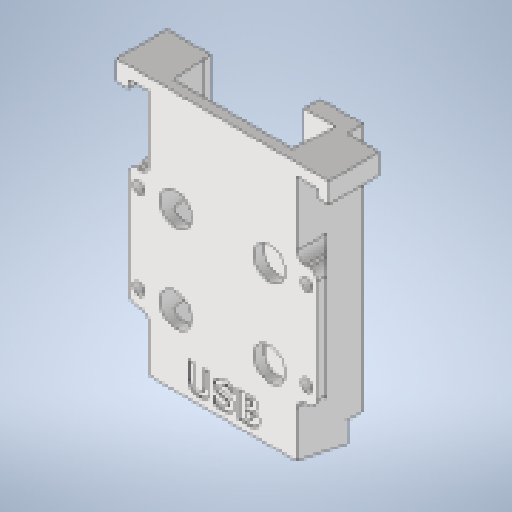
# Autodesk Inventor part: TPLink_holder
Saved by Autodesk Inventor 2025.1 (Build 291241000, 241)
## iProperties
Created: 2026-04-16
Part Number: TPLink_holder
Material: Generic
Document SubType Name: Modeling
Designer: User
Density: 1 g/cm^3
Appearance: Default
Author: User
## iProperties of the stored document TPLink_holder_3DPrint.ipt
Created: 2026-04-16
Part Number: TPLink_holder_3DPrint
Material: Generic
Document SubType Name: Modeling
Designer: User
Density: 1 g/cm^3
Appearance: Default
Author: User
Autodesk Inventor part; units mm, degrees
ref_plane "YZ Plane" through (0, 0, 0) normal (1, 0, 0) x (0, 1, 0)
ref_plane "XZ Plane" through (0, 0, 0) normal (0, 1, 0) x (-1, 0, 0)
ref_plane "XY Plane" through (0, 0, 0) normal (0, 0, 1) x (1, 0, 0)
sketch "Sketch1" plane through (0, 0, 0) normal (0, 0, 1) x (1, 0, 0)
  circle A0 centre (-2.95, 14.395506) radius 1.5
  circle A1 centre (-2.95, -16.594833) radius 1.5
  circle A2 centre (-31.617451, -2.998229) radius 1.5
  arc A3 (-69.05, 18.492691) -> (-67.05, 16.492691) centre (-67.05, 18.492691) ccw
  line L0 (-69.05, 18.492691) -> (-69.05, 32.5)
  line L1 (-69.05, 32.5) -> (-72.05, 32.5)
  line L2 (-72.05, -34) -> (-72.05, 32.5)
  line L3 (-72.05, -34) -> (-69.05, -34)
  line L4 (-69.05, -34) -> (-69.05, -28.3)
  arc A4 (-67.05, -26.3) -> (-69.05, -28.3) centre (-67.05, -28.3) ccw
  line L5 (-67.05, -26.3) -> (-43.236448, -26.3)
  arc A5 (-43.236448, -26.3) -> (-41.236448, -24.3) centre (-43.236448, -24.3) ccw
  line L6 (-41.236448, -24.3) -> (-41.236448, -18.699925)
  arc A6 (-39.236448, -16.699925) -> (-41.236448, -18.699925) centre (-39.236448, -18.699925) ccw
  line L7 (-39.236448, -16.699925) -> (-25.536448, -16.699925)
  arc A7 (-23.536448, -18.699925) -> (-25.536448, -16.699925) centre (-25.536448, -18.699925) ccw
  line L8 (-23.536448, -18.699925) -> (-23.536448, -24.3)
  arc A8 (-23.536448, -24.3) -> (-21.536448, -26.3) centre (-21.536448, -24.3) ccw
  line L9 (-21.536448, -26.3) -> (16.15, -26.3)
  line L10 (16.15, -26.3) -> (16.15, -32)
  line L11 (16.15, -32) -> (19.15, -32)
  line L12 (19.15, -32) -> (19.15, -23)
  line L13 (19.15, -23) -> (11.85, -23)
  line L14 (5.85, -17) -> (11.85, -23)
  line L15 (5.85, -17) -> (5.85, -14.65)
  arc A9 (5.85, -14.65) -> (3.85, -12.65) centre (3.85, -14.65) ccw
  line L16 (3.85, -12.65) -> (-0.35, -12.65)
  arc A10 (-2.35, -10.65) -> (-0.35, -12.65) centre (-0.35, -10.65) ccw
  line L17 (-2.35, -10.65) -> (-2.35, 10.65)
  arc A11 (-0.35, 12.65) -> (-2.35, 10.65) centre (-0.35, 10.65) ccw
  line L18 (-0.35, 12.65) -> (3.85, 12.65)
  arc A12 (3.85, 12.65) -> (5.85, 14.65) centre (3.85, 14.65) ccw
  line L19 (5.85, 14.65) -> (5.85, 17)
  line L20 (11.85, 23) -> (5.85, 17)
  line L21 (11.85, 23) -> (19.15, 23)
  line L22 (19.15, 23) -> (19.15, 32)
  line L23 (19.15, 32) -> (16.15, 32)
  line L24 (16.15, 32) -> (16.15, 24.50333)
  line L25 (16.15, 24.50333) -> (11.05, 24.50333)
  line L26 (11.05, 24.50333) -> (11.05, 25.3)
  line L27 (11.05, 25.3) -> (-13.742981, 25.3)
  arc A13 (-13.742981, 25.3) -> (-15.742981, 23.3) centre (-13.742981, 23.3) ccw
  line L28 (-15.742981, 23.3) -> (-15.742981, 17.729975)
  arc A14 (-17.742981, 15.729975) -> (-15.742981, 17.729975) centre (-17.742981, 17.729975) ccw
  line L29 (-17.742981, 15.729975) -> (-38.743552, 15.729975)
  arc A15 (-40.743552, 17.729975) -> (-38.743552, 15.729975) centre (-38.743552, 17.729975) ccw
  line L30 (-40.743552, 17.729975) -> (-40.743552, 23.3)
  arc A16 (-40.743552, 23.3) -> (-42.743552, 25.3) centre (-42.743552, 23.3) ccw
  line L31 (-42.743552, 25.3) -> (-50.436553, 25.3)
  arc A17 (-50.436553, 25.3) -> (-52.436553, 23.3) centre (-50.436553, 23.3) ccw
  line L32 (-52.436553, 23.3) -> (-52.436553, 18.492691)
  arc A18 (-54.436553, 16.492691) -> (-52.436553, 18.492691) centre (-54.436553, 18.492691) ccw
  line L33 (-54.436553, 16.492691) -> (-67.05, 16.492691)
  line L34 (-6.107274, -23.520089) -> (-6.107274, 44.519148)
  ellipse E0 centre (-12.125904, -23.420884) end of major axis (-9.966677, -29.178822) minor radius 6 (-12.028521, -29.552133) -> (-6.107274, -23.520089) ccw
  line L35 (-30.786028, -29.552133) -> (-12.028521, -29.552133)
  ellipse E1 centre (-30.688645, -23.420884) end of major axis (-32.847872, -29.178822) minor radius 6 (-36.707274, -23.520089) -> (-30.786028, -29.552133) ccw
  line L36 (-36.707274, 44.519148) -> (-36.707274, -23.520089)
  line L37 (-36.707274, -16.699925) -> (-36.707274, -14.699925)
  line L38 (-36.707274, -14.699925) -> (-6.107274, -14.699925)
  line L39 (-36.707274, 15.729975) -> (-36.707274, 13.729975)
  line L40 (-36.707274, 13.729975) -> (-6.107274, 13.729975)
  line L41 (-36.707274, -14.699925) -> (-6.107274, 13.729975)
  line L42 (-36.707274, 13.729975) -> (-6.107274, -14.699925)
  line L43 (-36.707274, -14.699925) -> (-33.044239, -11.296666)
  line L44 (-36.707274, 13.729975) -> (-33.044239, 10.326716)
  line L45 (-6.107274, -14.699925) -> (-9.77031, -11.296666)
  line L46 (-6.107274, 13.729975) -> (-9.77031, 10.326716)
  circle A19 centre (-9.77031, -11.296666) radius 1.5
  circle A20 centre (-9.77031, 10.326716) radius 1.5
  circle A21 centre (-33.044239, 10.326716) radius 1.5
  circle A22 centre (-33.044239, -11.296666) radius 1.5
  point P0 (0, 0)
  dimension "d0" = 2
  dimension "d1" = 90
  dimension "d2" = 2
  dimension "d3" = 5
  dimension "d4" = 5
  dimension "d5" = 5
  dimension "d6" = 5
  dimension "d7" = 3
  dimension "d8" = 3
  dimension "d9" = 3
  dimension "d10" = 3
  constraints: 20 end point, 13 point on line, 4 centre point, 3 coincident, 2 perpendicular, 2 other
  measures "d0" distance of L37.start L37.end
  measures "d1" angle of L37 L38
  measures "d2" distance of L39.start L39.end
  measures "d3" distance of L37.end L43.end
  measures "d4" distance of L39.end L44.end
  measures "d5" distance of L38.end L45.end
  measures "d6" distance of L40.end L46.end
  measures "d7" diameter of A19
  measures "d8" diameter of A20
  measures "d9" diameter of A21
  measures "d10" diameter of A22
extrude "Extrusion1" add sketch "Sketch1" along normal blind 4 contours A2 | L42 A21 L41 A22 L36 | L40 L41 A20 L42 A21 | L41 A22 L42 A19 L38 | L34 L42 A19 L41 A20
sketch "Sketch2" plane through (0, 0, 4) normal (0, 0, 1) x (1, 0, 0)
  circle A0 centre (-9.77031, -11.296666) radius 1.5
  circle A1 centre (-9.77031, 10.326716) radius 1.5
  circle A2 centre (-33.044239, -11.296666) radius 1.5
  circle A3 centre (-33.044239, 10.326716) radius 1.5
  circle A4 centre (-9.77031, -11.296666) radius 3.663035
  line L0 (-6.107274, -14.699925) -> (-6.107274, 13.729975)
  circle A5 centre (-9.77031, 10.326716) radius 3.677483
  circle A6 centre (-33.044239, 10.326716) radius 3.663035
  line L1 (-36.707274, 13.729975) -> (-36.707274, -14.699925)
  circle A7 centre (-33.044239, -11.296666) radius 3.663035
  line L2 (-36.707274, -14.699925) -> (-6.107274, -14.699925)
  line L3 (-6.107274, 13.729975) -> (-36.707274, 13.729975)
  point P0 (0, 0)
  point P1 (-34.399103, -14.699925)
  point P2 (-36.707274, -11.296666)
  point P3 (-34.399103, 13.729975)
  point P4 (-36.707274, 10.326716)
  point P5 (-6.107274, 10.001058)
  point P6 (-8.376858, 13.729975)
  point P7 (-6.107274, -11.296666)
  point P8 (-8.415446, -14.699925)
  constraints: 4 centre point, 4 coincident, 3 tangent
extrude "Extrusion2" cut sketch "Sketch2" against normal blind 2 contours A0 | A1 | A2 | A3 | A4 L2 | L0 L2 A4 | L2 A4 | A5 L3 L0 | L2 A7 | A7 L2 | A5 L3 L0 | A5 L3 | L2 L1 A7 | L3 A6 | A6 L3 | A6 L1 L3
sketch "Sketch3" plane through (-36.707274, -14.699925, 0) normal (-1, 0, 0) x (0, 0, 1)
  line L0 (4, 25.026641) -> (2, 25.026641)
  line L1 (2, 25.026641) -> (2, 28.4299)
  line L2 (0, 28.4299) -> (2, 28.4299)
  line L3 (0, 28.4299) -> (0, 0)
  line L4 (0, 0) -> (2, 0)
  line L5 (2, 0) -> (2, 3.403259)
  line L6 (4, 3.403259) -> (2, 3.403259)
  line L7 (4, 25.026641) -> (4, 3.403259)
  line L8 (0, 4.903259) -> (0, 1.903259)
  line L9 (4, 25.026641) -> (0, 25.026641)
  line L10 (0, 25.026641) -> (0, 3.403259)
  line L11 (0, 3.403259) -> (4, 3.403259)
  line L12 (4, 3.403259) -> (4, 25.026641)
  point P0 (0, 14.699925)
  point P1 (0, 3.403259)
  constraints: 8 end point, 2 parallel, 1 horizontal, 1 midpoint, 1 perpendicular
extrude "Extrusion3" add sketch "Sketch3" along normal blind 3
sketch "Sketch4" plane through (-6.107274, -14.699925, 0) normal (1, 0, 0) x (0, 0, -1)
  line L0 (-2, 28.4299) -> (-2, 24.700983)
  line L1 (-2, 24.700983) -> (-4, 24.700983)
  line L2 (-4, 3.403259) -> (-4, 24.700983)
  line L3 (-4, 3.403259) -> (-2, 3.403259)
  line L4 (-2, 3.403259) -> (-2, 0)
  line L5 (0, 0) -> (-2, 0)
  line L6 (0, 0) -> (0, 28.4299)
  line L7 (0, 28.4299) -> (-2, 28.4299)
  line L8 (-4, 3.403259) -> (0, 3.403259)
  line L9 (0, 3.403259) -> (0, 24.700983)
  line L10 (0, 24.700983) -> (-4, 24.700983)
  line L11 (-4, 24.700983) -> (-4, 3.403259)
  point P0 (0, 14.699925)
  constraints: 8 end point, 2 parallel, 1 horizontal, 1 perpendicular, 1 point on line
extrude "Extrusion4" add sketch "Sketch4" along normal blind 3
sketch "Sketch5" plane through (-39.707274, -11.296666, 4) normal (0, -1, 0) x (1, 0, 0)
  line L0 (3, 0) -> (3, -2) projected
  line L1 (3, 0) -> (0, 0) projected
  line L2 (0, -2) -> (0, 0) projected
  line L3 (3, -2) -> (0, -2) projected
  line L4 (33.6, 0) -> (33.6, -2) projected
  line L5 (33.6, -2) -> (36.6, -2) projected
  line L6 (36.6, 0) -> (36.6, -2) projected
  line L7 (33.6, 0) -> (36.6, 0) projected
  point P0 (39.707274, -4)
extrude "Extrusion5" add sketch "Sketch5" along normal up to surface (3.403259 mm away)
sketch "Sketch6" plane through (-6.107274, 10.001058, 4) normal (0, 1, 0) x (1, 0, 0)
  line L0 (0, 2) -> (0, 0) projected
  line L1 (0, 0) -> (3, 0) projected
  line L2 (3, 2) -> (3, 0) projected
  line L3 (0, 2) -> (3, 2) projected
  line L4 (-30.6, 0) -> (-30.6, 2) projected
  line L5 (-30.6, 2) -> (-33.6, 2) projected
  line L6 (-33.6, 0) -> (-33.6, 2) projected
  line L7 (-30.6, 0) -> (-33.6, 0) projected
  point P0 (6.107274, 4)
extrude "Extrusion6" add sketch "Sketch6" along normal up to surface (3.728917 mm away)
sketch "Sketch7" plane through (0, 0, 4) normal (0, 0, 1) x (1, 0, 0)
  line L0 (-39.707274, 13.729975) -> (-39.707274, -14.699925)
  line L1 (-3.107274, -14.699925) -> (-3.107274, 13.729975)
  line L2 (-3.107274, 13.729975) -> (-6.107274, 13.729975)
  line L3 (-3.107274, -14.699925) -> (-6.007274, -14.699925)
  line L4 (-6.007274, -14.699925) -> (-6.007274, 13.729975)
  line L5 (-6.007274, 13.729975) -> (-3.107274, 13.729975)
  line L6 (-3.107274, 13.729975) -> (-3.107274, -14.699925)
  line L7 (-39.707274, -14.699925) -> (-36.807274, -14.699925)
  line L8 (-36.807274, -14.699925) -> (-36.807274, 13.729975)
  line L9 (-36.807274, 13.729975) -> (-39.707274, 13.729975)
  line L10 (-39.707274, 13.729975) -> (-39.707274, -14.699925)
  point P0 (0, 0)
  dimension "d23" = 2.9
  dimension "d24" = 2.9
  constraints: 16 end point, 4 parallel, 2 horizontal, 2 perpendicular, 2 point on line
  measures "d23" distance of L4.end L5.end
  measures "d24" distance of L9.end L8.end
ref_plane "Work Plane1" through (-73.457274, -42.102133, 13.808489) normal (0, 0, 1) x (1, 0, 0)
extrude "Extrusion7" add sketch "Sketch7" along normal up to surface (9.808489 mm away)
sketch "Sketch8" plane through (-31.689375, -14.699925, 4) normal (0, -1, 0) x (1, 0, 0)
  line L0 (-4.267899, 9.808489) -> (-5.017899, 0.298489)
  line L1 (25.582101, 0.298489) -> (24.832101, 9.808489)
  line L2 (25.682101, 0) -> (25.682101, 9.808489)
  line L3 (-5.117899, 0) -> (-5.117899, 9.808489)
  line L4 (-4.46852, 9.808489) -> (-5.21728, 0.314213)
  line L5 (25.781482, 0.314213) -> (25.032722, 9.808489)
  line L6 (-8.017899, 9.808489) -> (-5.117899, 9.808489)
  line L7 (-5.117899, 9.808489) -> (-4.46852, 9.808489)
  line L8 (25.032722, 9.808489) -> (25.682101, 9.808489)
  point P0 (31.689375, -4)
  point P1 (25.682101, 1.574363)
  point P2 (-5.117899, 1.574363)
  dimension "d27" = 0.2
  dimension "d28" = 0.2
  constraints: 8 end point, 2 parallel, 1 collinear, 1 perpendicular
  measures "d27" distance between parallel lines of L0 L4
  measures "d28" distance between parallel lines of L1 L5
extrude "Extrusion8" add sketch "Sketch8" against normal up to surface (28.4299 mm away)
sketch "Sketch9" plane through (-3.107274, -14.699925, 13.808489) normal (0, 0, 1) x (1, 0, 0)
  line L0 (0, 0) -> (-3.549379, 0)
  line L1 (0, 28.4299) -> (0, 0)
  line L2 (0, 28.4299) -> (-3.549379, 28.4299)
  line L3 (-3.549379, 0) -> (-3.549379, 28.4299)
  line L4 (-36.6, 28.4299) -> (-33.050621, 28.4299)
  line L5 (-36.6, 0) -> (-36.6, 28.4299)
  line L6 (-33.050621, 0) -> (-36.6, 0)
  line L7 (-33.050621, 0) -> (-33.050621, 28.4299)
  point P0 (3.107274, 14.699925)
extrude "Extrusion9" add sketch "Sketch9" along normal blind 0.2
sketch "Sketch10" plane through (-3.107274, -14.699925, 14.008489) normal (0, 0, 1) x (1, 0, 0)
  line L0 (0, 0) -> (0, 28.4299) projected
  line L1 (-36.6, 28.4299) -> (-36.6, 0) projected
  line L2 (0, 0) -> (0, 28.4299) projected
  line L3 (0, 0) -> (-36.6, 0)
  line L4 (-36.6, 0) -> (-36.6, 28.4299)
  line L5 (-36.6, 28.4299) -> (0, 28.4299)
  line L6 (0, 28.4299) -> (0, 0)
  point P0 (3.107274, 14.699925)
  point P1 (-36.6, 0)
  constraints: 8 end point, 2 parallel, 1 horizontal, 1 perpendicular
extrude "Extrusion10" add sketch "Sketch10" along normal blind 2.5
sketch "Sketch11" plane through (-39.707274, -14.699925, 0) normal (-1, 0, 0) x (0, 0, 1)
  line L0 (4.298489, -14.852208) -> (13.808489, -12.852208)
  line L1 (4.339649, -15.047926) -> (13.849649, -13.047926)
  line L2 (16.508489, 28.4299) -> (16.508489, 0)
  line L3 (0, 0) -> (16.508489, 0)
  line L4 (0, -15.960576) -> (0, 0)
  line L5 (16.508489, 0) -> (16.508489, 28.4299)
  line L6 (16.508489, 11.085503) -> (16.508489, -12.488759)
  line L7 (16.508489, -12.488759) -> (0, -15.960576)
  point P0 (0, 14.699925)
  point P1 (4.339649, -15.047926)
  point P2 (13.849649, -13.047926)
  dimension "d35" = 0.2
  constraints: 8 end point, 1 collinear, 1 parallel, 1 point on line, 1 vertical
  measures "d35" distance between parallel lines of L0 L1
extrude "Extrusion11" add sketch "Sketch11" against normal up to surface surface through (-36.157895, -14.699925, 13.808489) normal (0.9969046, 0, -0.0786202)
sketch "Sketch12" plane through (-3.107274, -14.699925, 0) normal (1, 0, 0) x (0, 0, -1)
  line L0 (-16.508489, -12.488759) -> (-16.508489, 0)
  line L1 (0, -15.960576) -> (-16.508489, -12.488759)
  line L2 (0, 0) -> (0, -15.960576)
  line L3 (0, 0) -> (-16.508489, 0)
  point P0 (0, 14.699925)
extrude "Extrusion12" add sketch "Sketch12" against normal up to surface surface through (-6.007274, -14.699925, 5.574363) normal (-0.9969046, 0, -0.0786202)
sketch "Sketch13" plane through (-3.107274, -14.699925, 0) normal (1, 0, 0) x (0, 0, -1)
  line L0 (-16.508489, 28.4299) -> (-16.508489, -12.488759)
  line L1 (-14.008489, 0) -> (-14.008489, 28.4299)
  line L2 (-16.508489, -12.488759) -> (0, -15.960576)
  line L3 (-14.008489, 6.427758) -> (-14.008489, -13.014522)
  line L4 (-5.574363, 28.4299) -> (-13.808489, 28.4299)
  line L5 (-13.808489, 0) -> (-13.808489, 28.4299)
  line L6 (-14.008489, 0) -> (-13.808489, 0)
  line L7 (-16.508489, 0) -> (-14.008489, 0)
  line L8 (-16.508489, -12.488759) -> (-16.508489, 0)
  line L9 (0, -15.960576) -> (-16.508489, -12.488759)
  line L10 (0, 0) -> (0, -15.960576)
  line L11 (-5.574363, 0) -> (0, 0)
  line L12 (-5.574363, 28.4299) -> (-5.574363, 0)
  point P0 (0, 14.699925)
  constraints: 2 end point, 1 point on line, 1 vertical
extrude "Extrusion13" add sketch "Sketch13" against normal up to surface contours L7 L3 L2 L0 surface through (-36.157895, -14.699925, 13.808489) normal (0.9969046, 0, -0.0786202)
sketch "Sketch14" plane through (-31.689375, -14.699925, 4) normal (0, -1, 0) x (1, 0, 0)
  line L0 (26.12172, -4) -> (25.682101, 1.574363)
  line L1 (25.682101, 0) -> (25.682101, 1.574363)
  line L2 (25.582101, 0) -> (25.682101, 0)
  line L3 (25.582101, -2) -> (25.582101, 0)
  line L4 (25.582101, -2) -> (20.564202, -2)
  line L5 (20.564202, -2) -> (20.564202, 0)
  line L6 (0, 0) -> (20.564202, 0)
  line L7 (0, 0) -> (0, -2)
  line L8 (0, -2) -> (-5.017899, -2)
  line L9 (-5.017899, 0) -> (-5.017899, -2)
  line L10 (-5.117899, 0) -> (-5.017899, 0)
  line L11 (-5.117899, 0) -> (-5.117899, 1.574363)
  line L12 (-5.117899, 1.574363) -> (-5.557517, -4)
  line L13 (-5.557517, -4) -> (26.12172, -4)
  line L14 (-5.017899, 0) -> (-5.24206, 0)
  line L15 (25.582101, 0) -> (25.806262, 0)
  line L16 (20.564202, 0) -> (25.682101, 0)
  line L17 (-5.017899, 0) -> (2.308172, 0)
  line L18 (0, 0) -> (-5.017899, 0)
  point P0 (31.689375, -4)
  constraints: 8 end point, 3 point on line, 2 perpendicular, 1 horizontal
extrude "Extrusion14" add sketch "Sketch14" along normal up to surface contours L13 L12 L14 L10 L9 L8 L7 L6 L5 L4 L3 L2 L15 L0 | L3 L4 L5 L16 | L17 L7 L8 L9 surface through (-39.707274, -27.188684, 16.508489) normal (0, -0.9785934, 0.205803)
sketch "Sketch15" plane through (-3.107274, -14.699925, 0) normal (1, 0, 0) x (0, 0, -1)
  line L0 (-16.508489, -12.488759) -> (0, -15.960576)
  line L1 (-16.508489, -14.021572) -> (-0.308705, -17.428466)
  line L2 (-16.508489, 28.4299) -> (-16.508489, -12.488759)
  line L3 (0, -17.300075) -> (0, -8.300075)
  line L4 (0, -8.300075) -> (0, -17.493388)
  line L5 (0, -17.493388) -> (-16.508489, -14.021572)
  line L6 (-16.508489, -14.021572) -> (-16.508489, -12.488759)
  point P0 (0, 14.699925)
  point P1 (-0.308705, -17.428466)
  dimension "d44" = 1.5
  constraints: 8 end point, 2 parallel, 1 vertical
  measures "d44" distance between parallel lines of L0 L1
extrude "Extrusion15" add sketch "Sketch15" against normal blind 10
sketch "Sketch16" plane through (-39.707274, -14.699925, 0) normal (-1, 0, 0) x (0, 0, 1)
  line L0 (0, -17.493388) -> (16.508489, -14.021572)
  line L1 (16.508489, -14.021572) -> (16.508489, -12.488759)
  line L2 (14.008489, -13.014522) -> (16.508489, -12.488759)
  line L3 (14.008489, -13.014522) -> (4, -15.119356)
  line L4 (0, -15.960576) -> (4, -15.119356)
  line L5 (0, -15.960576) -> (0, -17.493388)
  point P0 (0, 14.699925)
extrude "Extrusion16" add sketch "Sketch16" against normal blind 10
sketch "Sketch17" plane through (-3.107274, -14.699925, 16.508489) normal (0, 0, 1) x (1, 0, 0)
  circle A0 centre (-6.663035, 3.403259) radius 1.5
  circle A1 centre (-29.936965, 3.403259) radius 1.5
  circle A2 centre (-29.936965, 3.403259) radius 4
  circle A3 centre (-6.663035, 3.403259) radius 4
  point P0 (3.107274, 14.699925)
  dimension "d49" = 8
  dimension "d50" = 8
  constraints: 2 centre point, 2 coincident
  measures "d49" diameter of A2
  measures "d50" diameter of A3
extrude "Extrusion17" cut sketch "Sketch17" against normal up to surface (2.5 mm away) contours A0 | A1 | A2 | A3
sketch "Sketch18" plane through (0, 0, 0) normal (0, 0, -1) x (-1, 0, 0)
  line L0 (23.536448, -18.699925) -> (23.536448, -24.3)
  arc A0 (21.536448, -26.3) -> (23.536448, -24.3) centre (21.536448, -24.3) ccw
  arc A1 (25.536448, -16.699925) -> (23.536448, -18.699925) centre (25.536448, -18.699925) ccw
  line L1 (39.236448, -16.699925) -> (25.536448, -16.699925)
  arc A2 (41.236448, -18.699925) -> (39.236448, -16.699925) centre (39.236448, -18.699925) ccw
  line L2 (21.536448, -26.3) -> (-16.15, -26.3)
  line L3 (39.707274, -32.193313) -> (29.707274, -32.193313)
  line L4 (39.707274, 13.729975) -> (39.707274, -32.193313)
  line L5 (29.707274, -30.660501) -> (13.107274, -30.660501)
  line L6 (29.707274, -32.193313) -> (29.707274, -30.660501)
  line L7 (13.107274, -30.660501) -> (13.107274, -32.193313)
  line L8 (3.107274, -32.193313) -> (13.107274, -32.193313)
  line L9 (3.107274, -32.193313) -> (3.107274, 13.729975)
  point P0 (0, 0)
  point P1 (3.107274, -26.3)
  point P2 (39.707274, -16.756134)
extrude "Extrusion18" cut sketch "Sketch18" against normal up to surface (4 mm away)
sketch "Sketch19" plane through (-39.707274, 13.729975, 0) normal (0, 1, 0) x (1, 0, 0)
  line L0 (3.549379, -13.808489) -> (3.549379, -14.008489)
  line L1 (2.9, -5.574363) -> (3.549379, -13.808489)
  line L2 (2.9, -4) -> (2.9, -5.574363)
  line L3 (3, -4) -> (2.9, -4)
  line L4 (3, -2) -> (3, -4)
  line L5 (8.017899, -2) -> (3, -2)
  line L6 (8.017899, -2) -> (8.017899, -4)
  line L7 (28.543513, -4) -> (8.017899, -4)
  line L8 (28.543513, -4) -> (28.543513, -2)
  line L9 (28.543513, -2) -> (33.6, -2)
  line L10 (33.6, -4) -> (33.6, -2)
  line L11 (33.7, -4) -> (33.6, -4)
  line L12 (33.7, -4) -> (33.7, -5.574363)
  line L13 (33.050621, -13.808489) -> (33.7, -5.574363)
  line L14 (33.050621, -13.808489) -> (33.050621, -14.008489)
  line L15 (33.050621, -14.008489) -> (3.549379, -14.008489)
  line L16 (0, 0) -> (0, -16.508489)
  line L17 (36.6, -16.508489) -> (0, -16.508489)
  line L18 (36.6, 0) -> (36.6, -16.508489)
  line L19 (0, 0) -> (36.6, 0)
  line L20 (33.6, -4) -> (26.259482, -4)
  line L21 (28.543513, -4) -> (33.6, -4)
  line L22 (3, -4) -> (3, -2)
  line L23 (8.017899, -4) -> (3, -4)
  point P0 (39.707274, 0)
  constraints: 4 end point, 1 collinear, 1 horizontal
ref_plane "Work Plane2" through (-13.742981, 25.3, -20) normal (0, 1, 0) x (0, 0, 1)
extrude "Extrusion19" add sketch "Sketch19" along normal up to surface (11.570025 mm away) contours L4 L5 L6 L23 | L20 L8 L9 L10 | L19 L18 L17 L16
sketch "Sketch20" plane through (0, 0, 0) normal (0, 0, -1) x (-1, 0, 0)
  circle A0 centre (33.044239, -11.296666) radius 1.5
  circle A1 centre (9.77031, -11.296666) radius 1.5
  circle A2 centre (9.77031, 10.326716) radius 1.5
  circle A3 centre (33.044239, 10.326716) radius 1.5
  line L0 (3.107274, -26.3) -> (21.536448, -26.3)
  arc A4 (21.536448, -26.3) -> (23.536448, -24.3) centre (21.536448, -24.3) ccw
  line L1 (23.536448, -24.3) -> (23.536448, -18.699925)
  arc A5 (25.536448, -16.699925) -> (23.536448, -18.699925) centre (25.536448, -18.699925) ccw
  line L2 (25.536448, -16.699925) -> (39.236448, -16.699925)
  arc A6 (39.707274, -16.756134) -> (39.236448, -16.699925) centre (39.236448, -18.699925) ccw
  line L3 (39.707274, -16.756134) -> (39.707274, 25.3)
  line L4 (39.707274, 25.3) -> (3.107274, 25.3)
  line L5 (3.107274, -26.3) -> (3.107274, 25.3)
  line L6 (17.742981, 15.729975) -> (38.743552, 15.729975)
  arc A7 (15.742981, 17.729975) -> (17.742981, 15.729975) centre (17.742981, 17.729975) ccw
  line L7 (15.742981, 23.3) -> (15.742981, 17.729975)
  arc A8 (15.742981, 23.3) -> (13.742981, 25.3) centre (13.742981, 23.3) ccw
  arc A9 (38.743552, 15.729975) -> (40.743552, 17.729975) centre (38.743552, 17.729975) ccw
  point P0 (0, 0)
  point P1 (39.707274, 15.97748)
extrude "Extrusion20" cut sketch "Sketch20" against normal up to surface (4 mm away) contours L4 L3 A9 L6 A7 L7 A8
sketch "Sketch21" plane through (-39.707274, 25.3, 16.508489) normal (0, 1, 0) x (1, 0, 0)
  line L0 (2.9, 12.508489) -> (0, 12.508489)
  line L1 (0, 0) -> (0, 12.508489)
  line L2 (36.6, 0) -> (0, 0)
  line L3 (36.6, 16.508489) -> (36.6, 0)
  line L4 (25.964293, 16.508489) -> (36.6, 16.508489)
  line L5 (25.964293, 12.508489) -> (25.964293, 16.508489)
  line L6 (33.7, 12.508489) -> (25.964293, 12.508489)
  line L7 (33.7, 10.934126) -> (33.7, 12.508489)
  line L8 (33.050621, 2.7) -> (33.7, 10.934126)
  line L9 (33.050621, 2.5) -> (33.050621, 2.7)
  line L10 (3.549379, 2.5) -> (33.050621, 2.5)
  line L11 (3.549379, 2.7) -> (3.549379, 2.5)
  line L12 (2.9, 10.934126) -> (3.549379, 2.7)
  line L13 (2.9, 12.508489) -> (2.9, 10.934126)
  point P0 (39.707274, 16.508489)
extrude "Extrusion21" add sketch "Sketch21" along normal blind 10
sketch "Sketch22" plane through (-3.107274, -14.699925, 16.508489) normal (0, 0, 1) x (1, 0, 0)
  arc A0 (-8.056487, 28.4299) -> (-3, 24.700983) centre (-6.663035, 25.026641) ccw
  arc A1 (-33.6, 25.026641) -> (-28.582101, 28.4299) centre (-29.936965, 25.026641) ccw
  circle A2 centre (-29.936965, 25.026641) radius 4
  circle A3 centre (-6.663035, 25.026641) radius 4
  point P0 (3.107274, 14.699925)
  dimension "d61" = 8
  dimension "d62" = 8
  constraints: 2 centre point, 2 coincident
  measures "d61" diameter of A2
  measures "d62" diameter of A3
extrude "Extrusion22" cut sketch "Sketch22" against normal up to surface (12.508489 mm away)
sketch "Sketch23" plane through (-13.107274, -14.699925, 0) normal (-1, 0, 0) x (0, 0, 1)
  line L0 (14.008489, -13.014522) -> (16.508489, -12.488759)
  line L1 (4, -16.652169) -> (16.508489, -14.021572)
  line L2 (16.508489, -14.021572) -> (16.508489, -12.488759)
  line L3 (14.008489, -13.014522) -> (14.008489, 0)
  line L4 (14.008489, -13.014522) -> (14.008489, -14.547334)
  point P0 (0, 14.699925)
  constraints: 2 end point, 1 collinear, 1 point on line
extrude "Extrusion23" add sketch "Sketch23" along normal up to surface (16.6 mm away)
sketch "Sketch24" plane through (-3.107274, -14.699925, 16.508489) normal (0, 0, 1) x (1, 0, 0)
  line L0 (-27.478748, -5.612028) -> (-8.934144, -5.612028) construction
  line L1 (-8.934144, -5.612028) -> (-8.934144, -12.418264) construction
  line L2 (-8.934144, -12.418264) -> (-27.478748, -12.418264) construction
  line L3 (-27.478748, -12.418264) -> (-27.478748, -5.612028) construction
  spline S0 degree 2 poles (-24.149957, -12.418264) (-25.471917, -12.418264) (-26.894749, -11.144086) (-26.894749, -9.91238) knots 0 0 0 1 2 2 2
  line L4 (-26.894749, -9.91238) -> (-26.894749, -5.728828)
  line L5 (-26.894749, -5.728828) -> (-25.248936, -5.728828)
  line L6 (-25.248936, -5.728828) -> (-25.248936, -9.816817)
  spline S1 degree 2 poles (-25.248936, -9.816817) (-25.248936, -10.501688) (-24.733955, -11.170631) (-24.149957, -11.170631) knots 0 0 0 1 2 2 2
  spline S2 degree 2 poles (-24.149957, -11.170631) (-23.581886, -11.170631) (-23.050978, -10.528233) (-23.050978, -9.816817) knots 0 0 0 1 2 2 2
  line L7 (-23.050978, -9.816817) -> (-23.050978, -5.728828)
  line L8 (-23.050978, -5.728828) -> (-21.405164, -5.728828)
  line L9 (-21.405164, -5.728828) -> (-21.405164, -9.907071)
  spline S3 degree 2 poles (-21.405164, -9.907071) (-21.405164, -11.117541) (-22.790833, -12.418264) (-24.149957, -12.418264) knots 0 0 0 1 2 2 2
  spline S4 degree 2 poles (-18.118846, -12.397028) (-18.872735, -12.397028) (-20.008877, -12.105029) (-20.497312, -11.892666) knots 0 0 0 1 2 2 2
  line L10 (-20.497312, -11.892666) -> (-20.497312, -10.331797)
  line L11 (-20.497312, -10.331797) -> (-20.348658, -10.331797)
  spline S5 degree 2 poles (-20.348658, -10.331797) (-19.854914, -10.751214) (-18.67099, -11.202486) (-18.113537, -11.202486) knots 0 0 0 1 2 2 2
  spline S6 degree 2 poles (-18.113537, -11.202486) (-17.970192, -11.202486) (-17.508302, -11.138777) (-17.370266, -11.075068) knots 0 0 0 1 2 2 2
  spline S7 degree 2 poles (-17.370266, -11.075068) (-17.200376, -11.000741) (-16.961467, -10.729978) (-16.961467, -10.512306) knots 0 0 0 1 2 2 2
  spline S8 degree 2 poles (-16.961467, -10.512306) (-16.961467, -10.262779) (-17.34903, -9.954853) (-17.614484, -9.885835) knots 0 0 0 1 2 2 2
  spline S9 degree 2 poles (-17.614484, -9.885835) (-17.948955, -9.79558) (-18.708153, -9.641617) (-19.042625, -9.524818) knots 0 0 0 1 2 2 2
  spline S10 degree 2 poles (-19.042625, -9.524818) (-19.801823, -9.259364) (-20.460149, -8.351512) (-20.460149, -7.67195) knots 0 0 0 1 2 2 2
  spline S11 degree 2 poles (-20.460149, -7.67195) (-20.460149, -6.75348) (-18.904589, -5.612028) (-17.736592, -5.612028) knots 0 0 0 1 2 2 2
  spline S12 degree 2 poles (-17.736592, -5.612028) (-17.152594, -5.612028) (-15.995215, -5.850937) (-15.538635, -6.052682) knots 0 0 0 1 2 2 2
  line L12 (-15.538635, -6.052682) -> (-15.538635, -7.549841)
  line L13 (-15.538635, -7.549841) -> (-15.68198, -7.549841)
  spline S13 degree 2 poles (-15.68198, -7.549841) (-16.048306, -7.236606) (-17.099503, -6.80657) (-17.651647, -6.80657) knots 0 0 0 1 2 2 2
  spline S14 degree 2 poles (-17.651647, -6.80657) (-17.869319, -6.80657) (-18.2091, -6.870279) (-18.400227, -6.955225) knots 0 0 0 1 2 2 2
  spline S15 degree 2 poles (-18.400227, -6.955225) (-18.55419, -7.024243) (-18.777171, -7.300314) (-18.777171, -7.470205) knots 0 0 0 1 2 2 2
  spline S16 degree 2 poles (-18.777171, -7.470205) (-18.777171, -7.725041) (-18.421463, -8.01704) (-17.911792, -8.13384) knots 0 0 0 1 2 2 2
  spline S17 degree 2 poles (-17.911792, -8.13384) (-17.582629, -8.208167) (-16.972085, -8.351512) (-16.621686, -8.47362) knots 0 0 0 1 2 2 2
  spline S18 degree 2 poles (-16.621686, -8.47362) (-15.942124, -8.723147) (-15.27849, -9.551363) (-15.27849, -10.230925) knots 0 0 0 1 2 2 2
  spline S19 degree 2 poles (-15.27849, -10.230925) (-15.27849, -11.207795) (-16.812813, -12.397028) (-18.118846, -12.397028) knots 0 0 0 1 2 2 2
  spline S20 degree 2 poles (-9.199597, -10.273397) (-9.199597, -10.761832) (-9.571233, -11.499794) (-9.879159, -11.744012) knots 0 0 0 1 2 2 2
  spline S21 degree 2 poles (-9.879159, -11.744012) (-10.250794, -12.036011) (-11.132101, -12.280228) (-11.816972, -12.280228) knots 0 0 0 1 2 2 2
  line L14 (-11.816972, -12.280228) -> (-14.434347, -12.280228)
  line L15 (-14.434347, -12.280228) -> (-14.434347, -5.728828)
  line L16 (-14.434347, -5.728828) -> (-12.124898, -5.728828)
  spline S22 degree 2 poles (-12.124898, -5.728828) (-11.402864, -5.728828) (-10.659593, -5.840318) (-10.33574, -6.015518) knots 0 0 0 1 2 2 2
  spline S23 degree 2 poles (-10.33574, -6.015518) (-9.980032, -6.201336) (-9.634942, -6.838425) (-9.634942, -7.252533) knots 0 0 0 1 2 2 2
  spline S24 degree 2 poles (-9.634942, -7.252533) (-9.634942, -7.73035) (-10.112758, -8.478929) (-10.537485, -8.654129) knots 0 0 0 1 2 2 2
  line L17 (-10.537485, -8.654129) -> (-10.537485, -8.685983)
  spline S25 degree 2 poles (-10.537485, -8.685983) (-9.926941, -8.813401) (-9.199597, -9.604454) (-9.199597, -10.273397) knots 0 0 0 1 2 2 2
  spline S26 degree 2 poles (-10.898502, -10.246852) (-10.898502, -9.938926) (-11.142719, -9.593836) (-11.386937, -9.503581) knots 0 0 0 1 2 2 2
  spline S27 degree 2 poles (-11.386937, -9.503581) (-11.535591, -9.445181) (-12.06119, -9.434563) (-12.496534, -9.434563) knots 0 0 0 1 2 2 2
  line L18 (-12.496534, -9.434563) -> (-12.799151, -9.434563)
  line L19 (-12.799151, -9.434563) -> (-12.799151, -11.085686)
  line L20 (-12.799151, -11.085686) -> (-12.708897, -11.085686)
  spline S28 degree 2 poles (-12.708897, -11.085686) (-12.071808, -11.085686) (-11.583373, -11.069759) (-11.328537, -10.958268) knots 0 0 0 1 2 2 2
  spline S29 degree 2 poles (-11.328537, -10.958268) (-11.105556, -10.857396) (-10.898502, -10.48576) (-10.898502, -10.246852) knots 0 0 0 1 2 2 2
  spline S30 degree 2 poles (-11.307301, -7.576386) (-11.307301, -7.417114) (-11.471882, -7.082642) (-11.641773, -7.008315) knots 0 0 0 1 2 2 2
  spline S31 degree 2 poles (-11.641773, -7.008315) (-11.801045, -6.933988) (-12.247007, -6.92337) (-12.687661, -6.92337) knots 0 0 0 1 2 2 2
  line L21 (-12.687661, -6.92337) -> (-12.799151, -6.92337)
  line L22 (-12.799151, -6.92337) -> (-12.799151, -8.314348)
  line L23 (-12.799151, -8.314348) -> (-12.592097, -8.314348)
  spline S32 degree 2 poles (-12.592097, -8.314348) (-12.17268, -8.314348) (-11.832899, -8.298421) (-11.652391, -8.213476) knots 0 0 0 1 2 2 2
  spline S33 degree 2 poles (-11.652391, -8.213476) (-11.455955, -8.117912) (-11.307301, -7.794059) (-11.307301, -7.576386) knots 0 0 0 1 2 2 2
  point P0 (3.107274, 14.699925)
  constraints: 2 other
emboss "Emboss1" sketch "Sketch24" operation cut depth 0.5 direction (0, 0, -1)
sketch "Sketch25" plane through (-3.107274, -14.699925, 16.508489) normal (0, 0, 1) x (1, 0, 0)
  line L0 (0, 49.999925) -> (0, -14.021572)
  line L1 (-36.6, -14.021572) -> (-36.6, 49.999925)
  circle A0 centre (-6.663035, 3.403259) radius 4
  circle A1 centre (-6.663035, 25.026641) radius 4
  line L2 (0, -11.600075) -> (0, 49.999925)
  line L3 (0, 25.026641) -> (-5, 25.026641)
  line L4 (0, 25.026641) -> (5, 25.026641)
  line L5 (-6.663035, 3.403259) -> (0, 3.403259)
  line L6 (0, 3.403259) -> (5, 3.403259)
  circle A2 centre (2.5, 25.026641) radius 1.5
  circle A3 centre (2.5, 3.403259) radius 1.5
  line L7 (5, 3.403259) -> (5, 25.026641)
  line L8 (5, 21.026641) -> (0, 21.026641)
  line L9 (0, 21.026641) -> (0, 29.026641)
  line L10 (0, 29.026641) -> (5, 29.026641)
  line L11 (5, 29.026641) -> (5, 21.026641)
  line L12 (5, 21.026641) -> (0, 29.026641) construction
  line L13 (0, 21.026641) -> (5, 29.026641) construction
  line L14 (5, -0.596741) -> (0, -0.596741)
  line L15 (0, -0.596741) -> (0, 7.403259)
  line L16 (0, 7.403259) -> (5, 7.403259)
  line L17 (5, 7.403259) -> (5, -0.596741)
  line L18 (5, -0.596741) -> (0, 7.403259) construction
  line L19 (0, -0.596741) -> (5, 7.403259) construction
  point P0 (3.107274, 14.699925)
  point P1 (0, 29.026641)
  point P2 (0, -0.596741)
  point P3 (5, 3.403259)
  dimension "d69" = 5
  dimension "d70" = 5
  dimension "d71" = 5
  dimension "d72" = 3
  dimension "d73" = 3
  dimension "d74" = 8
  dimension "d75" = 8
  constraints: 34 end point, 6 midpoint, 6 point on line, 4 parallel, 4 perpendicular, 2 centre point, 2 horizontal
  measures "d69" distance of L3.start L3.end
  measures "d70" distance of L3.start L4.end
  measures "d71" distance of L5.end L6.end
  measures "d72" diameter of A2
  measures "d73" diameter of A3
  measures "d74" distance of L8.end L9.end
  measures "d75" distance of L14.end L15.end
extrude "Extrusion24" add sketch "Sketch25" against normal blind 2.5 contours L10 L11 L4 A2 L0 | L4 A2 L7 L8 L0 | L8 L7 L16 L0 | L16 L7 L6 A3 L0 | L6 A3 L17 L14 L0
sketch "Sketch26" plane through (-3.107274, 14.326716, 16.508489) normal (0, 1, 0) x (1, 0, 0)
  line L0 (0, 2.5) -> (5, 2.5)
  line L1 (0, 2.5) -> (0, 7.5)
  line L2 (0, 0) -> (0, 12.508489)
  line L3 (5, 0) -> (5, 2.5)
  line L4 (0, 7.5) -> (5, 2.5)
  point P0 (3.107274, 16.508489)
  dimension "d78" = 5
  constraints: 4 end point, 1 point on line
  measures "d78" distance of L0.start L1.end
extrude "Extrusion25" add sketch "Sketch26" against normal up to surface (29.623382 mm away)
sketch "Sketch27" plane through (-3.107274, -14.699925, 16.508489) normal (0, 0, 1) x (1, 0, 0)
  circle A0 centre (2.5, 25.026641) radius 1.5
  circle A1 centre (2.5, 3.403259) radius 1.5
  point P0 (3.107274, 14.699925)
extrude "Extrusion26" cut sketch "Sketch27" against normal through all
fillet "Fillet1" radius 2 4 edges at (-3.1073, -15.2967, 12.7585) (1.8927, -15.2967, 15.2585) (1.8927, 14.3267, 15.2585) (-3.1073, 14.3267, 12.7585)
sketch "Sketch28" plane through (-3.107274, -14.699925, 16.508489) normal (0, 0, 1) x (1, 0, 0)
  circle A0 centre (-29.936965, 3.403259) radius 4
  circle A1 centre (-29.936965, 25.026641) radius 4
  line L0 (-29.936965, 25.026641) -> (-36.6, 25.026641)
  line L1 (-36.6, -14.021572) -> (-36.6, 49.999925)
  circle A2 centre (-29.936965, 3.403259) radius 1.5
  line L2 (-29.936965, 3.403259) -> (-36.6, 3.403259)
  line L3 (-36.6, 3.403259) -> (-41.6, 3.403259)
  line L4 (-36.6, 25.026641) -> (-41.6, 25.026641)
  line L5 (-41.6, 25.026641) -> (-41.6, 3.403259)
  circle A3 centre (-39.1, 3.403259) radius 1.5
  circle A4 centre (-39.1, 25.026641) radius 1.5
  line L6 (-36.6, 7.403259) -> (-41.6, 7.403259)
  line L7 (-41.6, 7.403259) -> (-41.6, -0.596741)
  line L8 (-41.6, -0.596741) -> (-36.6, -0.596741)
  line L9 (-36.6, -0.596741) -> (-36.6, 7.403259)
  line L10 (-36.6, 7.403259) -> (-41.6, -0.596741) construction
  line L11 (-41.6, 7.403259) -> (-36.6, -0.596741) construction
  line L12 (-36.6, 29.026641) -> (-41.6, 29.026641)
  line L13 (-41.6, 29.026641) -> (-41.6, 21.026641)
  line L14 (-41.6, 21.026641) -> (-36.6, 21.026641)
  line L15 (-36.6, 21.026641) -> (-36.6, 29.026641)
  line L16 (-36.6, 29.026641) -> (-41.6, 21.026641) construction
  line L17 (-41.6, 29.026641) -> (-36.6, 21.026641) construction
  point P0 (3.107274, 14.699925)
  point P1 (-36.6, 29.026641)
  point P2 (-41.6, 25.026641)
  point P3 (-36.6, -0.596741)
  dimension "d84" = 5
  dimension "d85" = 5
  dimension "d86" = 3
  dimension "d87" = 3
  dimension "d88" = 8
  dimension "d89" = 5
  dimension "d90" = 8
  constraints: 34 end point, 6 midpoint, 5 horizontal, 4 parallel, 3 perpendicular, 2 centre point, 2 point on line
  measures "d84" distance of L2.end L3.end
  measures "d85" distance of L0.end L4.end
  measures "d86" diameter of A3
  measures "d87" diameter of A4
  measures "d88" distance of L7.end L6.end
  measures "d89" distance of L14.end L13.end
  measures "d90" distance of L13.end L12.end
extrude "Extrusion27" add sketch "Sketch28" against normal blind 2.5 contours L8 L7 L3 A3 L1 | L3 A3 L5 L6 L1 | L6 L5 L14 L1 | L14 L5 L4 A4 L1 | L4 A4 L13 L12 L1
sketch "Sketch29" plane through (-44.707274, -15.296666, 16.508489) normal (0, -1, 0) x (1, 0, 0)
  line L0 (5, -2.5) -> (0, -2.5)
  line L1 (5, -12.508489) -> (5, 0)
  line L2 (5, -2.5) -> (5, -7.5)
  line L3 (5, -7.5) -> (0, -2.5)
  point P0 (44.707274, -16.508489)
  dimension "d93" = 5
  constraints: 4 end point, 1 point on line
  measures "d93" distance of L0.start L2.end
extrude "Extrusion28" add sketch "Sketch29" against normal up to surface (29.623382 mm away)
sketch "Sketch30" plane through (-3.107274, -14.699925, 16.508489) normal (0, 0, 1) x (1, 0, 0)
  circle A0 centre (-39.1, 25.026641) radius 1.5
  circle A1 centre (-39.1, 3.403259) radius 1.5
  point P0 (3.107274, 14.699925)
extrude "Extrusion29" cut sketch "Sketch30" against normal blind 10
fillet "Fillet2" radius 2 4 edges at (-39.7073, 14.3267, 12.7585) (-44.7073, 14.3267, 15.2585) (-44.7073, -15.2967, 15.2585) (-39.7073, -15.2967, 12.7585)
sketch "Sketch31" plane through (-3.107274, -14.699925, 16.508489) normal (0, 0, 1) x (1, 0, 0)
  line L0 (-36.6, 49.999925) -> (0, 49.999925)
  line L1 (-36.6, 46.999925) -> (0, 46.999925)
  line L2 (0, 46.999925) -> (5, 46.999925)
  line L3 (5, 46.999925) -> (5, 49.999925)
  line L4 (5, 49.999925) -> (0, 49.999925)
  line L5 (0, 49.999925) -> (0, 46.999925)
  line L6 (-36.6, 46.999925) -> (-41.6, 46.999925)
  line L7 (-41.6, 46.999925) -> (-41.6, 49.999925)
  line L8 (-41.6, 49.999925) -> (-36.6, 49.999925)
  line L9 (-36.6, 49.999925) -> (-36.6, 46.999925)
  line L10 (5, 49.999925) -> (8, 49.999925)
  line L11 (8, 49.999925) -> (8, 44.999925)
  line L12 (8, 44.999925) -> (5, 44.999925)
  line L13 (5, 44.999925) -> (5, 49.999925)
  line L14 (-41.6, 49.999925) -> (-44.6, 49.999925)
  line L15 (-44.6, 49.999925) -> (-44.6, 44.999925)
  line L16 (-44.6, 44.999925) -> (-41.6, 44.999925)
  line L17 (-41.6, 44.999925) -> (-41.6, 49.999925)
  point P0 (3.107274, 14.699925)
  point P1 (-41.6, 46.999925)
  dimension "d99" = 3
  dimension "d100" = 5
  dimension "d101" = 5
  dimension "d102" = 3
  dimension "d103" = 5
  dimension "d104" = 3
  dimension "d105" = 5
  constraints: 34 end point, 9 parallel, 4 horizontal, 4 perpendicular, 1 point on line
  measures "d99" distance between parallel lines of L0 L1
  measures "d100" distance of L4.end L3.end
  measures "d101" distance of L7.end L8.end
  measures "d102" distance of L11.end L12.end
  measures "d103" distance of L10.end L11.end
  measures "d104" distance of L16.end L15.end
  measures "d105" distance of L15.end L14.end
extrude "Extrusion30" add sketch "Sketch31" against normal up to surface (12.508489 mm away) contours L9 L6 L7 L8 | L4 L3 L2 L5 | L7 L17 L16 L15 L14 | L10 L11 L12 L13 L3
sketch "Sketch32" plane through (-3.107274, -14.699925, 16.508489) normal (0, 0, 1) x (1, 0, 0)
  circle A0 centre (-6.663035, 3.403259) radius 4
  circle A1 centre (-29.936965, 3.403259) radius 4
  point P0 (3.107274, 14.699925)
extrude "Extrusion31" cut sketch "Sketch32" against normal up to surface (12.508489 mm away)
equation "\"d51\" = d49"
body "Solid1"
